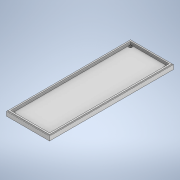
# Autodesk Inventor part: top
Saved by Autodesk Inventor 2022.2 (Build 262287000, 287)
## iProperties
Created: 2021-12-16
Part Number: top
Material: Generic
Document SubType Name: Modeling
Designer: samlo
Density: 1 g/cm^3
Appearance: Default
Author: samlo
Autodesk Inventor part; units mm, degrees
ref_plane "YZ Plane" through (0, 0, 0) normal (1, 0, 0) x (0, 1, 0)
ref_plane "XZ Plane" through (0, 0, 0) normal (0, 1, 0) x (-1, 0, 0)
ref_plane "XY Plane" through (0, 0, 0) normal (0, 0, 1) x (1, 0, 0)
sketch "Sketch1" plane through (0, 0, 0) normal (0, 1, 0) x (-1, 0, 0)
  line L0 (0, 0) -> (61, 0)
  line L1 (61, 0) -> (61, -176)
  line L2 (61, -176) -> (0, -176)
  line L3 (0, -176) -> (0, 0)
  dimension "d0" = 176
  dimension "d1" = 61
  constraints: 8 end point, 2 parallel, 1 horizontal, 1 perpendicular
  measures "d0" distance of L2.end L0.start
  measures "d1" distance of L0.start L0.end
extrude "Extrusion1" add sketch "Sketch1" along normal blind 3
sketch "Sketch2" plane through (0, 3, 0) normal (0, 1, 0) x (1, 0, 0)
  line L0 (0, 0) -> (0, 176) projected
  line L1 (0, 176) -> (-61, 176) projected
  line L2 (0, 0) -> (-61, 0)
  line L3 (-61, 0) -> (-61, 176)
  line L4 (-61, 176) -> (0, 176)
  line L5 (0, 176) -> (0, 0)
  line L6 (-3, 3) -> (-58, 3)
  line L7 (-58, 3) -> (-58, 173)
  line L8 (-58, 173) -> (-3, 173)
  line L9 (-3, 173) -> (-3, 3)
  dimension "d4" = 3
  dimension "d5" = 3
  dimension "d6" = 3
  dimension "d7" = 3
  constraints: 16 end point, 4 parallel, 2 horizontal, 2 perpendicular
  measures "d4" distance between parallel lines of L3 L7
  measures "d5" distance between parallel lines of L1 L8
  measures "d6" distance between parallel lines of L0 L9
  measures "d7" distance between parallel lines of L6 L2
extrude "Extrusion2" add sketch "Sketch2" along normal blind 4
sketch "Sketch3" plane through (0, 3, 0) normal (0, 1, 0) x (1, 0, 0)
  circle A0 centre (-5.5, 5.5) radius 2
  line L0 (-3, 3) -> (-58, 3) projected
  line L1 (-3, 173) -> (-3, 3) projected
  circle A1 centre (-55.5, 5.5) radius 2
  line L2 (-58, 3) -> (-58, 173) projected
  circle A2 centre (-55.5, 170.5) radius 2
  circle A3 centre (-5.5, 170.5) radius 2
  line L3 (-58, 173) -> (-3, 173) projected
  point P0 (0, 0)
  dimension "d10" = 4
  dimension "d11" = 2.5
  dimension "d12" = 2.5
  dimension "d15" = 4
  dimension "d16" = 2.5
  dimension "d17" = 2.5
  dimension "d18" = 4
  dimension "d19" = 4
  dimension "d20" = 2.5
  dimension "d21" = 2.5
  dimension "d22" = 2.5
  dimension "d23" = 2.5
  constraints: 4 centre point
  measures "d10" diameter of A0
  measures "d11" distance from line of L0 A0.centre
  measures "d12" distance from line of L1 A0.centre
  measures "d15" diameter of A1
  measures "d16" distance from line of L2 A1.centre
  measures "d17" distance from line of L0 A1.centre
  measures "d18" diameter of A2
  measures "d19" diameter of A3
  measures "d20" distance from line of L1 A3.centre
  measures "d21" distance from line of L3 A3.centre
  measures "d22" distance from line of L3 A2.centre
  measures "d23" distance from line of L2 A2.centre
extrude "Extrusion3" cut sketch "Sketch3" against normal blind 10 contours A0 | A1 | A2 | A3
lip "Lip1" kind groove height 1 width 1 edges at (-61, 7, -88) (-30.5, 7, 0) (0, 7, -88) (-30.5, 7, -176) guide face at (-60, 7, -116.3333)
body "Solid1"
